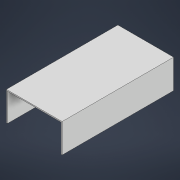
# Autodesk Inventor part: Ebene3_mitte_vorne
Saved by Autodesk Inventor 2021 (Build 250183000, 183)
## iProperties
Created: 2021-02-07
Part Number: Ebene3_mitte_vorne
Material: Generisch
Document SubType Name: Modeling
Designer: laure
Density: 1 g/cm^3
Appearance: Vorgabe
Author: laure
Autodesk Inventor part; units mm, degrees
ref_plane "YZ Plane" through (0, 0, 0) normal (1, 0, 0) x (0, 1, 0)
ref_plane "XZ Plane" through (0, 0, 0) normal (0, 1, 0) x (-1, 0, 0)
ref_plane "XY Plane" through (0, 0, 0) normal (0, 0, 1) x (1, 0, 0)
sketch "Skizze1" plane through (0, 0, 0) normal (0, 1, 0) x (-1, 0, 0)
  line L0 (50, -100) -> (-50, -100)
  line L1 (-50, -100) -> (-50, 100)
  line L2 (-50, 100) -> (50, 100)
  line L3 (50, 100) -> (50, -100)
  line L4 (0, -140) -> (0, 140) projected
  line L5 (70, 0) -> (-70, 0) projected
  point P0 (0, 0)
  dimension "d0" = 100
  dimension "d1" = 200
  constraints: 8 end point, 2 parallel, 1 horizontal, 1 perpendicular, 2 other
  measures "d0" distance between parallel lines of L1 L3
  measures "d1" distance between parallel lines of L2 L0
extrude "Extrusion1" add sketch "Skizze1" along normal mid plane 2
sketch "Skizze2" plane through (0, -1, 0) normal (0, -1, 0) x (1, 0, 0)
  line L0 (50, 100) -> (50, -100) projected
  line L1 (50, -100) -> (-50, -100) projected
  line L2 (50, 100) -> (48, 100)
  line L3 (48, 100) -> (48, -100)
  line L4 (48, -100) -> (50, -100)
  line L5 (50, -100) -> (50, 100)
  line L6 (-50, -100) -> (-50, 100) projected
  line L7 (-50, 100) -> (-48, 100)
  line L8 (-48, 100) -> (-48, -100)
  line L9 (-48, -100) -> (-50, -100)
  line L10 (-50, -100) -> (-50, 100)
  point P0 (0, 0)
  dimension "d4" = 2
  dimension "d5" = 2
  constraints: 16 end point, 4 parallel, 2 horizontal, 2 perpendicular, 2 point on line
  measures "d4" distance of L4.end L3.end
  measures "d5" distance of L8.end L9.end
extrude "Extrusion2" add sketch "Skizze2" along normal blind 50
